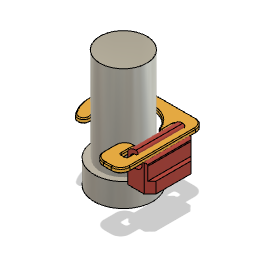
Rail Dog Clip (Autodesk Fusion 360 design; units mm, degrees)
Autodesk Fusion 360 part; units mm, degrees
sketch "Profile" plane through (0, 0, 0) normal (0, 0, 1) x (1, 0, 0) in component "Rail Dog"
  line L0 (0, 0) -> (12, 0)
  line L1 (12, 0) -> (12, 4.75)
  line L2 (12, 4.75) -> (0, 4.75)
  line L3 (0, 4.75) -> (0, 0)
  line L4 (1.75, 4.75) -> (10.25, 4.75)
  line L5 (10.25, 4.75) -> (10.25, 10.25)
  line L6 (10.25, 10.25) -> (1.75, 10.25)
  line L7 (1.75, 10.25) -> (1.75, 4.75)
  circle A0 centre (6, 10.25) radius 4.25
  circle A1 centre (6, 10.25) radius 2.6
  circle A2 centre (6.0188, 13.6749) radius 0.825
  circle A3 centre (9.3988, 10.6728) radius 0.825
  dimension "d1" = 12
  dimension "d2" = 4.75
  dimension "d3" = 8.5
  dimension "d4" = 5.5
  dimension "d5" = 5.2
  constraint horizontal L0
  constraint vertical L1
  constraint vertical L3
  constraint coincident L0.start L3.end
  constraint horizontal L4
  constraint vertical L5
  constraint horizontal L6
  constraint vertical L7
  constraint coincident L2 L4.start
  constraint coincident L5.end A0
  constraint tangent L5 A0
  constraint coincident L6.end A0
  constraint midpoint L2 L4
  constraint concentric A0 A1
  constraint tangent A0 A2
  constraint tangent A0 A3
  measures "d1" distance of L0.start L0.end
  measures "d2" distance of L0.start L2.end
  measures "d3" distance of L5.end L6.end
  measures "d4" distance of L4.start L6.end
  measures "d5" diameter of A1
extrude "Extrude1" add sketch "Profile" along normal blind 20 contours L0 L1 L2 L3 L4 | L2 L4 L5 L7 A0 | L6 A0 A1 A2 | L6 A0 A1 A3 | L6 A0 A3 | A2 | L6 A3 | L6 A3 | L6 A1 A3 makes body 1 in component "Rail Dog"
sketch "Sketch1" plane through (0, 0, 0) normal (0, 1, 0) x (1, 0, 0) in component "Parf Dog"
  circle A0 centre (0, 0) radius 12.5
  circle A1 centre (0, 0) radius 10
  dimension "d10" = 25
  dimension "d11" = 20
  constraint coincident A0.centre A1.centre
  constraint concentric A0 A1
  measures "d10" diameter of A0
  measures "d11" diameter of A1
extrude "Extrude2" add sketch "Sketch1" along normal blind 50 separate body contours A1 makes body 2 in component "Parf Dog"
extrude "Extrude1'" add sketch "Sketch1" along normal blind 10 separate body contours A0 | A1 makes body 3 in component "Parf Dog"
sketch "Profile (2)" plane through (0, 0, 0) normal (0, 1, 0) x (1, 0, 0) in component "Spring Clip"
  line L0 (-11.8766, -28) -> (-11.8766, 8) construction
  line L1 (7.4234, 8) -> (7.4234, -28) construction
  line L2 (6.0234, 0) -> (6.0234, -20) construction
  line L3 (-9.8766, -21) -> (-9.8766, 8) construction
  line L4 (-11.8766, 3) -> (-9.8766, 3)
  line L5 (-11.8766, -17) -> (-9.8766, -17)
  line L6 (0.9234, 1.5) -> (3.4234, 1.5)
  line L7 (3.4234, 1.5) -> (3.4234, -21.5)
  line L8 (3.4234, -21.5) -> (0.9234, -21.5)
  line L9 (0.9234, -21.5) -> (0.9234, 1.5)
  line L10 (7.4234, 8) -> (7.4234, -28)
  line L11 (0.1234, -10) -> (0.1234, -25)
  line L12 (-3.8766, -28) -> (-3.8766, -15)
  line L13 (48.2225, -10) -> (-36.1758, -10) construction
  line L14 (-11.8766, 8) -> (7.4234, 8)
  line L15 (-11.8766, -28) -> (7.4234, -28)
  arc A0 (-11.8766, 3) -> (-11.8766, -17) centre (-11.8766, -7) ccw
  arc A1 (-9.8766, -17) -> (-9.8766, 3) centre (-9.8766, -7) ccw
  circle A2 centre (-21.8766, -14.5) radius 2.5
  line L16 (-0.3373, -4) -> (0.9234, -4)
  line L17 (-3.8766, -15) -> (0.9234, -15)
  line L18 (1.75, 0) -> (6.0234, 0)
  line L19 (1.75, -20) -> (6.0234, -20)
  arc A3 (-11.8766, 8) -> (-23.8766, -16) centre (-11.8766, -7) ccw
  point P0 (-22.0766, -10)
  point P1 (-16.9925, -12.7499)
  dimension "d55" = 2
  dimension "d64" = 12.8
  dimension "d69" = 23
  dimension "d70" = 10
  dimension "d71" = 10
  dimension "d72" = 36
  dimension "d73" = 4
  dimension "d74" = 2.6
  dimension "d75" = 2.5
  dimension "d77" = 10
  dimension "d81" = 8
  dimension "d82" = 4
  dimension "d84" = 5
  dimension "d85" = 5
  dimension "d86" = 4
  constraint coincident L0 L4.start
  constraint coincident L3 L4.end
  constraint coincident L0 L5.start
  constraint coincident L3 L5.end
  constraint horizontal L6
  constraint vertical L7
  constraint horizontal L8
  constraint vertical L9
  constraint perpendicular L2 L13
  constraint midpoint L2 L13
  constraint tangent L4 A0
  constraint tangent L4 A1
  constraint tangent L5 A1
  constraint symmetric L6 L8 L13
  constraint tangent A0 A2
  constraint coincident A1 L16.start
  constraint coincident L9 L16.end
  constraint perpendicular L9 L16
  constraint coincident A1 L12.end
  constraint coincident L9 L17.end
  constraint perpendicular L9 L17
  constraint vertical L11
  constraint tangent L11 A1
  constraint coincident L12.end L17.start
  constraint coincident L12.start L15
  constraint perpendicular L12 L15
  constraint coincident A2 A3.end
  constraint tangent L14 A3
  constraint tangent A2 A3
  measures "d55" distance of L0 L3
  measures "d64" distance of L0 L9
  measures "d69" distance of L6 L8
  measures "d70" radius of A0
  measures "d71" radius of A1
  measures "d72" distance of L14 L15
  measures "d73" distance of L7 L10
  measures "d74" distance of L2 L7
  measures "d75" distance of L7 L9
  measures "d77" distance of L0 A2.centre
  measures "d81" distance of L14 L18
  measures "d82" distance of L16 L18
  measures "d84" distance of L4 L14
  measures "d85" diameter of A2
  measures "d86" distance of L11 L12
extrude "Extrude1''" add sketch "Profile (2)" along normal blind 2 separate body contours L4 L6 L7 L8 L9 L10 L12 L14 L15 A0 A1 A2 L16 L17 A3 | A2 makes body 4 in component "Spring Clip"
fillet "Fillet5" radius 0.5 7 edges at (0.9234, 1, -1.5) (3.4234, 1, -1.5) (3.4234, 1, 21.5) (0.9234, 1, 21.5) (0.9234, 1, 15) (0.9234, 1, 4) (-0.3373, 1, 4) on bodies 4 in component "Spring Clip"
fillet "Fillet5" radius 4 4 edges at (7.4234, 1, 28) (7.4234, 1, -8) (-3.8766, 1, 28) (-3.8766, 1, 15) on bodies 4 in component "Spring Clip"
chamfer "Chamfer1" distance 0.4 angle 45 54 edges at (6.2518, 0, 26.8284) (7.4234, 0, 10) (6.2518, 0, -6.8284) (-4.2266, 0, -8) (-25.2931, 0, 0.2918) (-20.3766, 0, 16.5) (-20.8209, 0, 2.5279) (-10.8766, 0, -3) (-4.1031, 0, -1.165) (-0.2658, 0, 3.9082) (0.2231, 0, 4) (0.7769, 0, 3.8536) (0.9234, 0, 1.25) (1.0698, 0, -1.3536) (2.1734, 0, -1.5) (3.2769, 0, -1.3536) (3.4234, 0, 10) (3.2769, 0, 21.3536) (2.1734, 0, 21.5) (1.0698, 0, 21.3536) (0.9234, 0, 18.25) (0.7769, 0, 15.1464) (0.2734, 0, 15) (-2.7051, 0, 16.1716) (-3.8766, 0, 21.5) (-2.7051, 0, 26.8284) (1.7734, 0, 28) (-3.8766, 2, 21.5) (-2.7051, 2, 16.1716) (0.2734, 2, 15) (0.7769, 2, 15.1464) (0.9234, 2, 18.25) (1.0698, 2, 21.3536) (2.1734, 2, 21.5) (3.2769, 2, 21.3536) (3.4234, 2, 10) (3.2769, 2, -1.3536) (2.1734, 2, -1.5) (1.0698, 2, -1.3536) (0.9234, 2, 1.25) (0.7769, 2, 3.8536) (0.2231, 2, 4) (-0.2658, 2, 3.9082) (-4.1031, 2, -1.165) (-10.8766, 2, -3) (-20.8209, 2, 2.5279) (-20.3766, 2, 16.5) (-25.2931, 2, 0.2918) (-4.2266, 2, -8) (6.2518, 2, -6.8284) (7.4234, 2, 10) (6.2518, 2, 26.8284) (1.7734, 2, 28) (-2.7051, 2, 26.8284) on bodies 4 in component "Spring Clip"
chamfer "Chamfer1'" distance 2.5 angle 45 4 edges at (12, 2.375, 20) (0, 2.375, 20) (12, 2.375, 0) (0, 2.375, 0) on bodies 1 in component "Rail Dog"
component "Spring Clip" placed x (1, 0, 0) y (0, 1, 0) z (0, 0, 1) at (14, 11.3, -10)
component "Rail Dog" placed x (1, 0, 0) y (0, 1, 0) z (0, 0, 1) at (14, 2, -10)
component "Parf Dog" placed x (1, 0, 0) y (0, 1, 0) z (0, 0, 1) at (1.6, -12, 0)
named bodies: "UpBody"
